Autodesk Inventor part; units mm, degrees
(part 3 of 4)
  line L522 (9.5, 12.75) -> (20, 12.75)
  line L523 (20, 12.75) -> (20, -5.25)
  line L524 (20, -5.25) -> (9.5, -5.25)
  line L525 (9.5, -5.25) -> (9.5, 12.75)
  line L526 (9.5, 17.25) -> (20, 17.25)
  line L527 (20, 17.25) -> (20, 35.25)
  line L528 (20, 35.25) -> (9.5, 35.25)
  line L529 (9.5, 35.25) -> (9.5, 17.25)
  line L530 (9.5, 57.75) -> (20, 57.75)
  line L531 (20, 57.75) -> (20, 39.75)
  line L532 (20, 39.75) -> (9.5, 39.75)
  line L533 (9.5, 39.75) -> (9.5, 57.75)
  line L534 (9.5, 62.25) -> (20, 62.25)
  line L535 (20, 62.25) -> (20, 80.25)
  line L536 (20, 80.25) -> (9.5, 80.25)
  line L537 (9.5, 80.25) -> (9.5, 62.25)
  line L538 (9.5, 117.75) -> (20, 117.75)
  line L539 (20, 117.75) -> (20, 99.75)
  line L540 (20, 99.75) -> (9.5, 99.75)
  line L541 (9.5, 99.75) -> (9.5, 117.75)
  line L542 (9.5, 84.75) -> (20, 84.75)
  line L543 (20, 84.75) -> (20, 95.25)
  line L544 (20, 95.25) -> (9.5, 95.25)
  line L545 (9.5, 95.25) -> (9.5, 84.75)
  point P0 (0, 0)
  point P1 (9.5, -64.25)
  point P2 (20, -53.75)
  point P3 (20, -49.25)
  point P4 (20, -8.75)
  point P5 (20, -4.25)
  point P6 (20, 36.25)
  point P7 (9.5, 40.75)
  point P8 (20, 51.25)
  point P9 (20, 55.75)
  point P10 (20, 96.25)
  point P11 (20, 100.75)
  point P12 (35, 27.75)
  point P13 (35, 17.25)
  point P14 (39.5, 17.25)
  point P15 (39.5, 27.75)
  point P16 (35, 42.75)
  point P17 (35, 57.75)
  point P18 (35, 72.75)
  point P19 (35, -47.25)
  point P20 (35, -77.25)
  point P21 (35, -32.25)
  point P22 (39.5, -32.25)
  point P23 (35, -17.25)
  point P24 (39.5, -17.25)
  point P25 (39.5, -12.75)
  point P26 (39.5, -2.25)
  point P27 (35, 12.75)
  point P28 (35, 2.25)
  point P29 (39.5, 2.25)
  point P30 (39.5, 12.75)
  point P31 (9.5, 99.75)
  point P32 (20, 99.75)
  point P33 (20, 102.75)
  point P34 (20, 107.25)
  point P35 (9.5, 107.25)
  point P36 (9.5, 102.75)
  point P37 (9.5, 95.25)
  point P38 (9.5, 92.25)
  point P39 (9.5, 87.75)
  point P40 (20, 84.75)
  point P41 (20, 87.75)
  point P42 (20, 92.25)
  point P43 (9.5, 80.25)
  point P44 (9.5, 77.25)
  point P45 (9.5, 72.75)
  point P46 (20, 72.75)
  point P47 (20, 77.25)
  point P48 (9.5, 39.75)
  point P49 (20, 42.75)
  point P50 (20, 47.25)
  point P51 (9.5, 47.25)
  point P52 (9.5, 42.75)
  point P53 (20, 35.25)
  point P54 (9.5, 35.25)
  point P55 (9.5, 32.25)
  point P56 (9.5, 27.75)
  point P57 (20, 27.75)
  point P58 (20, 32.25)
  point P59 (9.5, -5.25)
  point P60 (20, -5.25)
  point P61 (20, -2.25)
  point P62 (20, 2.25)
  point P63 (9.5, 2.25)
  point P64 (9.5, -2.25)
  point P65 (9.5, -9.75)
  point P66 (9.5, -12.75)
  point P67 (9.5, -17.25)
  point P68 (20, -20.25)
  point P69 (20, -17.25)
  point P70 (20, -12.75)
  point P71 (9.5, -24.75)
  point P72 (9.5, -27.75)
  point P73 (9.5, -32.25)
  point P74 (20, -32.25)
  point P75 (20, -27.75)
  point P76 (9.5, -65.25)
  point P77 (20, -62.25)
  point P78 (20, -57.75)
  point P79 (9.5, -57.75)
  point P80 (9.5, -62.25)
  point P81 (9.5, -69.75)
  point P82 (9.5, -72.75)
  point P83 (9.5, -77.25)
  point P84 (20, -77.25)
  point P85 (20, -72.75)
  dimension "d223" = 0.25
  dimension "d224" = 10.5
  dimension "d225" = 10.5
  dimension "d226" = 0.25
  dimension "d229" = 15
  dimension "d232" = 15
  dimension "d283" = 10.5
  dimension "d284" = 18
  dimension "d285" = 18
  dimension "d286" = 18
  dimension "d287" = 10.5
  dimension "d288" = 4.5
  dimension "d289" = 18
  dimension "d290" = 18
  dimension "d291" = 18
  dimension "d292" = 18
  dimension "d293" = 18
  dimension "d294" = 10.5
  dimension "d295" = 4.5
  constraints: 1088 end point, 50 parallel, 26 horizontal, 25 perpendicular, 21 point on line, 2 collinear, 1 vertical, 886 other
  measures "d223" distance between parallel lines of L4 L0
  measures "d224" distance of L0.start L0.end
  measures "d225" distance of L0.end L1.end
  measures "d226" distance between parallel lines of L5 L3
  measures "d229" distance of L0.start L6.start
  measures "d232" distance of L0.start L66.start
  measures "d283" distance of L508.end L507.end
  measures "d284" distance of L507.end L506.end
  measures "d285" distance of L510.end L511.end
  measures "d286" distance of L514.end L515.end
  measures "d287" distance of L518.end L519.end
  measures "d288" distance between parallel lines of L516 L518
  measures "d289" distance of L522.end L523.end
  measures "d290" distance of L526.end L527.end
  measures "d291" distance of L530.end L531.end
  measures "d292" distance of L534.end L535.end
  measures "d293" distance of L538.end L539.end
  measures "d294" distance of L542.end L543.end
  measures "d295" distance between parallel lines of L536 L542
extrude "Extrusion8" add sketch "Sketch21" along normal blind 1 contours L0 L1 L2 L3 | L6 L7 L8 L9 | L66 L67 L68 L69 | L70 L71 L72 L73 | L130 L131 L132 L133 | L134 L135 L136 L137 | L162 L163 L164 L165 | L166 L167 L168 L169 | L170 L171 L172 L173 | L174 L175 L176 L177 | L178 L179 L180 L181 | L182 L183 L184 L185 | L186 L187 L188 L189 | L190 L191 L192 L193 | L194 L195 L196 L197 | L198 L199 L200 L201 | L226 L227 L228 L229 | L230 L231 L232 L233 | L234 L235 L236 L237 | L238 L239 L240 L241 | L242 L243 L244 L245 | L246 L247 L248 L249 | L250 L251 L252 L253 | L254 L255 L256 L257 | L258 L259 L260 L261 | L262 L263 L264 L265 | L266 L267 L268 L269 | L268 L509 L270 L507 | L270 L271 L508 L273 | L512 L271 L272 L273 | L272 L513 L274 L511 | L274 L275 L276 L277 | L278 L279 L280 L281 | L280 L517 L282 L515 | L282 L283 L516 L285 | L518 L283 L284 L285 | L284 L521 L286 L519 | L286 L287 L520 L289 | L524 L287 L288 L289 | L288 L525 L290 L523 | L290 L291 L292 L293 | L294 L295 L296 L297 | L296 L529 L298 L527 | L298 L299 L528 L301 | L532 L299 L300 L301 | L300 L533 L302 L531 | L302 L303 L304 L305 | L306 L307 L308 L309 | L308 L537 L310 L535 | L310 L311 L536 L313 | L542 L311 L312 L313 | L312 L545 L314 L543 | L314 L315 L544 L317 | L540 L315 L316 L317 | L316 L541 L318 L539 | L318 L319 L320 L321 | L322 L323 L324 L325 | L326 L327 L328 L329 | L330 L331 L332 L333 | L333 L452 L395 L450 | L395 L396 L397 L394 | L334 L335 L336 L337 | L337 L456 L399 L454 | L399 L400 L401 L398 | L338 L339 L340 L341 | L341 L460 L403 L458 | L403 L404 L405 L402 | L342 L343 L344 L345 | L345 L464 L407 L462 | L407 L408 L409 L406 | L346 L347 L348 L349 | L349 L468 L411 L466 | L411 L412 L413 L410 | L350 L351 L352 L353 | L353 L472 L415 L470 | L415 L416 L417 L414 | L354 L355 L356 L357 | L357 L476 L419 L474 | L419 L420 L421 L418 | L358 L359 L360 L361 | L361 L480 L423 L478 | L423 L424 L425 L422 | L362 L363 L364 L365 | L365 L484 L427 L482 | L427 L428 L429 L426 | L366 L367 L368 L369 | L369 L488 L431 L486 | L431 L432 L433 L430 | L370 L371 L372 L373 | L373 L492 L435 L490 | L435 L436 L437 L434 | L374 L375 L376 L377 | L377 L496 L439 L494 | L439 L440 L441 L438 | L378 L379 L380 L381 | L381 L500 L443 L498 | L443 L444 L445 L442 | L382 L383 L384 L385 | L385 L504 L447 L502 | L447 L448 L449 L446 | L386 L387 L388 L389 | L390 L391 L392 L393
sketch "Sketch23" plane through (0, 4, 0) normal (0, 1, 0) x (1, 0, 0)
  circle A0 centre (-63.5, -131.25) radius 10.25
  line L0 (-60.5, 128.25) -> (-60.5, -128.25) projected
  line L1 (-60.5, -128.25) -> (60.5, -128.25) projected
  circle A1 centre (63.5, 131.25) radius 10.25
  circle A2 centre (63.5, -131.25) radius 10.25
  line L2 (60.5, -128.25) -> (60.5, 128.25) projected
  line L3 (60.5, 128.25) -> (-60.5, 128.25) projected
  circle A3 centre (-63.5, 131.25) radius 10.25
  circle A4 centre (-63.5, 0) radius 7.75
  circle A5 centre (63.5, 0) radius 7.75
  point P0 (0, 0)
  point P1 (-53.6989, -128.25)
  point P2 (-60.5, -121.4489)
  dimension "d338" = 20.5
  dimension "d339" = 3
  dimension "d340" = 3
  dimension "d341" = 20.5
  dimension "d342" = 3
  dimension "d343" = 3
  dimension "d344" = 20.5
  dimension "d345" = 3
  dimension "d346" = 3
  dimension "d347" = 3
  dimension "d348" = 3
  dimension "d349" = 20.5
  dimension "d350" = 15.5
  dimension "d351" = 3
  dimension "d352" = 128.25
  dimension "d353" = 15.5
  dimension "d354" = 3
  dimension "d355" = 128.25
  constraints: 6 centre point
  measures "d338" diameter of A0
  measures "d339" distance from line of L0 A0.centre
  measures "d340" distance from line of A0.centre L1
  measures "d341" diameter of A2
  measures "d342" distance from line of L2 A2.centre
  measures "d343" distance from line of L1 A2.centre
  measures "d344" diameter of A1
  measures "d345" distance from line of L3 A1.centre
  measures "d346" distance from line of L2 A1.centre
  measures "d347" distance from line of L0 A3.centre
  measures "d348" distance from line of L3 A3.centre
  measures "d349" diameter of A3
  measures "d350" diameter of A4
  measures "d351" distance from line of L0 A4.centre
  measures "d352" distance from line of L3 A4.centre
  measures "d353" diameter of A5
  measures "d354" distance from line of L2 A5.centre
  measures "d355" distance from line of L1 A5.centre
extrude "Extrusion9" cut sketch "Sketch23" against normal through all contours L1 L0 A0 | A2 L2 L1 | L1 L2 A2 | A4 L0 | L0 A4 | A5 L2 | L2 A5 | A3 L3 L0 | L0 L3 A3 | L2 L3 A1 | A1 L3 L2 picked at (-59.7398, -124.0546)
sketch "Sketch24" plane through (0, 4, 0) normal (0, 1, 0) x (1, 0, 0)
  line L0 (-52, 0.5) -> (-23, 0.5)
  line L1 (-23, 0.5) -> (-23, 29.5) construction
  line L2 (-23, 29.5) -> (-52, 29.5)
  line L3 (-52, 29.5) -> (-52, 0.5) construction
  line L4 (-52, 30.5) -> (-23, 30.5)
  line L5 (-23, 30.5) -> (-23, 59.5)
  line L6 (-23, 59.5) -> (-52, 59.5)
  line L7 (-52, 59.5) -> (-52, 30.5)
  line L8 (-52, 60.5) -> (-23, 60.5)
  line L9 (-23, 60.5) -> (-23, 89.5)
  line L10 (-23, 89.5) -> (-52, 89.5)
  line L11 (-52, 89.5) -> (-52, 60.5)
  line L12 (-52, 90.5) -> (-23, 90.5)
  line L13 (-23, 90.5) -> (-23, 119.5)
  line L14 (-23, 119.5) -> (-52, 119.5)
  line L15 (-52, 119.5) -> (-52, 90.5)
  line L16 (-60.5, 121.4489) -> (-60.5, 7.1458) projected
  line L17 (-43.5, 9) -> (-31.5, 9) construction
  line L18 (-31.5, 9) -> (-31.5, 21) construction
  line L19 (-31.5, 21) -> (-43.5, 21) construction
  line L20 (-43.5, 21) -> (-43.5, 9)
  line L21 (-43.5, 39) -> (-31.5, 39)
  line L22 (-31.5, 39) -> (-31.5, 51)
  line L23 (-31.5, 51) -> (-43.5, 51)
  line L24 (-43.5, 51) -> (-43.5, 39)
  line L25 (-43.5, 69) -> (-31.5, 69)
  line L26 (-31.5, 69) -> (-31.5, 81)
  line L27 (-31.5, 81) -> (-43.5, 81)
  line L28 (-43.5, 81) -> (-43.5, 69)
  line L29 (-43.5, 99) -> (-31.5, 99)
  line L30 (-31.5, 99) -> (-31.5, 111)
  line L31 (-31.5, 111) -> (-43.5, 111)
  line L32 (-43.5, 111) -> (-43.5, 99)
  line L33 (-49.7, 0.1) -> (-43.5, 0.1)
  line L34 (-43.5, 0.1) -> (-43.5, 26.3)
  line L35 (-43.5, 26.3) -> (-49.7, 26.3)
  line L36 (-49.7, 26.3) -> (-49.7, 0.1)
  line L37 (-49.7, 30.1) -> (-43.5, 30.1)
  line L38 (-43.5, 30.1) -> (-43.5, 56.3)
  line L39 (-43.5, 56.3) -> (-49.7, 56.3)
  line L40 (-49.7, 56.3) -> (-49.7, 30.1)
  line L41 (-49.7, 60.1) -> (-43.5, 60.1)
  line L42 (-43.5, 60.1) -> (-43.5, 86.3)
  line L43 (-43.5, 86.3) -> (-49.7, 86.3)
  line L44 (-49.7, 86.3) -> (-49.7, 60.1)
  line L45 (-49.7, 90.1) -> (-43.5, 90.1)
  line L46 (-43.5, 90.1) -> (-43.5, 116.3)
  line L47 (-43.5, 116.3) -> (-49.7, 116.3)
  line L48 (-49.7, 116.3) -> (-49.7, 90.1)
  line L49 (-31.5, 26.3) -> (-27.5, 26.3)
  line L50 (-27.5, 26.3) -> (-27.5, 6.3)
  line L51 (-27.5, 6.3) -> (-31.5, 6.3)
  line L52 (-31.5, 6.3) -> (-31.5, 26.3)
  line L53 (-31.5, 36.3) -> (-27.5, 36.3)
  line L54 (-27.5, 36.3) -> (-27.5, 56.3)
  line L55 (-27.5, 56.3) -> (-31.5, 56.3)
  line L56 (-31.5, 56.3) -> (-31.5, 36.3)
  line L57 (-31.5, 66.3) -> (-27.5, 66.3)
  line L58 (-27.5, 66.3) -> (-27.5, 86.3)
  line L59 (-27.5, 86.3) -> (-31.5, 86.3)
  line L60 (-31.5, 86.3) -> (-31.5, 66.3)
  line L61 (-31.5, 96.3) -> (-27.5, 96.3)
  line L62 (-27.5, 96.3) -> (-27.5, 116.3)
  line L63 (-27.5, 116.3) -> (-31.5, 116.3)
  line L64 (-31.5, 116.3) -> (-31.5, 96.3)
  line L65 (53.6989, 128.25) -> (-53.6989, 128.25) projected
  point P0 (0, 0)
  point P1 (-49.7, 90.5)
  point P2 (-43.5, 90.5)
  point P3 (-43.5, 111)
  point P4 (-49.7, 60.5)
  point P5 (-43.5, 60.5)
  point P6 (-43.5, 69)
  point P7 (-43.5, 81)
  point P8 (-49.7, 30.5)
  point P9 (-43.5, 30.5)
  point P10 (-43.5, 9)
  point P11 (-31.5, 39)
  point P12 (-31.5, 81)
  point P13 (-31.5, 111)
  dimension "d358" = 29
  dimension "d359" = 29
  dimension "d360" = 29
  dimension "d361" = 29
  dimension "d362" = 29
  dimension "d363" = 29
  dimension "d364" = 29
  dimension "d365" = 8.5
  dimension "d366" = 1
  dimension "d367" = 1
  dimension "d368" = 1
  dimension "d370" = 12
  dimension "d371" = 12
  dimension "d372" = 12
  dimension "d373" = 12
  dimension "d374" = 12
  dimension "d375" = 8.5
  dimension "d376" = 8.5
  dimension "d377" = 8.5
  dimension "d378" = 8.5
  dimension "d379" = 8.5
  dimension "d380" = 6.2
  dimension "d381" = 0
  dimension "d382" = 26.2
  dimension "d383" = 5.3
  dimension "d384" = 6.2
  dimension "d385" = 26.2
  dimension "d386" = 5.3
  dimension "d387" = 6.2
  dimension "d388" = 0
  dimension "d389" = 26.2
  dimension "d390" = 5.3
  dimension "d391" = 0
  dimension "d392" = 6.2
  dimension "d393" = 26.2
  dimension "d394" = 5.3
  dimension "d397" = 5.3
  dimension "d398" = 20
  dimension "d399" = 4
  dimension "d400" = 0
  dimension "d401" = 4
  dimension "d402" = 20
  dimension "d403" = 20
  dimension "d404" = 20
  dimension "d405" = 5.3
  dimension "d406" = 5.3
  dimension "d407" = 5.3
  dimension "d408" = 0
  dimension "d422" = 8.75
  constraints: 128 end point, 32 parallel, 16 horizontal, 16 perpendicular, 15 point on line
  measures "d358" distance of L0.end L1.end
  measures "d359" distance of L1.end L2.end
  measures "d360" distance of L5.end L6.end
  measures "d361" distance of L4.end L5.end
  measures "d362" distance of L8.end L9.end
  measures "d363" distance of L13.end L14.end
  measures "d364" distance of L12.end L13.end
  measures "d365" distance between parallel lines of L16 L3
  measures "d366" distance between parallel lines of L2 L4
  measures "d367" distance between parallel lines of L6 L8
  measures "d368" distance between parallel lines of L10 L12
  measures "d370" distance of L19.end L17.start
  measures "d371" distance of L18.end L19.end
  measures "d372" distance of L23.end L21.start
  measures "d373" distance of L27.end L25.start
  measures "d374" distance of L31.end L29.start
  measures "d375" distance between parallel lines of L3 L20
  measures "d376" distance between parallel lines of L2 L19
  measures "d377" distance between parallel lines of L4 L21
  measures "d378" distance between parallel lines of L8 L25
  measures "d379" distance between parallel lines of L12 L29
  measures "d380" distance of L34.end L35.end
  measures "d381" distance between parallel lines of L20 L34
  measures "d382" distance of L35.end L33.start
  measures "d383" distance between parallel lines of L19 L35
  measures "d384" distance of L46.end L47.end
  measures "d385" distance of L39.end L37.start
  measures "d386" distance between parallel lines of L39 L23
  measures "d387" distance of L38.end L39.end
  measures "d388" distance between parallel lines of L24 L38
  measures "d389" distance of L41.end L42.end
  measures "d390" distance between parallel lines of L27 L43
  measures "d391" distance between parallel lines of L28 L42
  measures "d392" distance of L42.end L43.end
  measures "d393" distance of L47.end L45.start
  measures "d394" distance between parallel lines of L31 L47
  measures "d397" distance between parallel lines of L19 L49
  measures "d398" distance of L49.end L50.end
  measures "d399" distance of L49.start L49.end
  measures "d400" distance between parallel lines of L18 L52
  measures "d401" distance of L54.end L55.end
  measures "d402" distance of L53.end L54.end
  measures "d403" distance of L57.end L58.end
  measures "d404" distance of L61.end L62.end
  measures "d405" distance between parallel lines of L31 L63
  measures "d406" distance between parallel lines of L27 L59
  measures "d407" distance between parallel lines of L23 L55
  measures "d408" distance between parallel lines of L22 L56
  measures "d422" distance between parallel lines of L65 L14
extrude "Extrusion10" add sketch "Sketch24" along normal blind 2.4 contours L36 L35 L34 L20 L0 | L0 L34 L33 L36 | L40 L39 L38 L24 L4 | L22 L56 L55 L54 L53 | L44 L43 L42 L28 L8 | L26 L60 L59 L58 L57 | L48 L47 L46 L32 L12 | L30 L64 L63 L62 L61 | L49 L50 L51 L52
sketch "Sketch25" plane through (0, 6.4, 0) normal (0, 1, 0) x (1, 0, 0)
  circle A0 centre (-46.15, 3.9) radius 1.5 projected
  circle A1 centre (-46.15, 20.6) radius 1.5 projected
  circle A2 centre (-46.15, 33.9) radius 1.5 projected
  circle A3 centre (-46.15, 50.6) radius 1.5 projected
  circle A4 centre (-46.15, 63.9) radius 1.5 projected
  circle A5 centre (-46.15, 80.6) radius 1.5 projected
  circle A6 centre (-46.15, 93.9) radius 1.5 projected
  circle A7 centre (-46.15, 110.6) radius 1.5 projected
  point P0 (0, 0)
  constraints: 8 coincident
hole "Hole1" at (-46.15, 6.4, -33.9) at (-46.15, 6.4, -50.6) at (-46.15, 6.4, -20.6) at (-46.15, 6.4, -3.9) at (-46.15, 6.4, -63.9) at (-46.15, 6.4, -80.6) at (-46.15, 6.4, -93.9) at (-46.15, 6.4, -110.6) direction (0, -1, 0) diameter 2.6 end through all
sketch "Sketch27" plane through (0, 4, 0) normal (0, 1, 0) x (1, 0, 0)
  line L0 (-43.5, 0.1) -> (-43.5, 26.3) projected
  line L1 (-27.5, 6.3) -> (-27.5, 26.3) projected
  line L2 (-43.5, 0.1) -> (-27.5, 0.1)
  line L3 (-27.5, 0.1) -> (-27.5, 6.3)
  line L4 (-27.5, 6.3) -> (-43.5, 6.3)
  line L5 (-43.5, 6.3) -> (-43.5, 0.1)
  line L6 (-43.5, 30.5) -> (-43.5, 56.3) projected
  line L7 (-27.5, 36.3) -> (-27.5, 56.3) projected
  line L8 (-43.5, 30.5) -> (-27.5, 30.5)
  line L9 (-27.5, 30.5) -> (-27.5, 36.3)
  line L10 (-27.5, 36.3) -> (-43.5, 36.3)
  line L11 (-43.5, 36.3) -> (-43.5, 30.5)
  line L12 (-43.5, 60.5) -> (-43.5, 86.3) projected
  line L13 (-31.5, 66.3) -> (-27.5, 66.3) projected
  line L14 (-43.5, 60.5) -> (-27.5, 60.5)
  line L15 (-27.5, 60.5) -> (-27.5, 66.3)
  line L16 (-27.5, 66.3) -> (-43.5, 66.3)
  line L17 (-43.5, 66.3) -> (-43.5, 60.5)
  line L18 (-43.5, 90.5) -> (-43.5, 116.3) projected
  line L19 (-31.5, 96.3) -> (-27.5, 96.3) projected
  line L20 (-43.5, 90.5) -> (-27.5, 90.5)
  line L21 (-27.5, 90.5) -> (-27.5, 96.3)
  line L22 (-27.5, 96.3) -> (-43.5, 96.3)
  line L23 (-43.5, 96.3) -> (-43.5, 90.5)
  line L24 (-60.5, 121.4489) -> (-60.5, 7.1458) projected
  line L25 (53.6989, 128.25) -> (-53.6989, 128.25) projected
  line L26 (-60.5, 120.75) -> (-19.75, 120.75)
  line L27 (-19.75, 120.75) -> (-19.75, 128.25)
  line L28 (-19.75, 128.25) -> (-60.5, 128.25)
  line L29 (-60.5, 128.25) -> (-60.5, 120.75)
  line L30 (-52.75, 123.75) -> (-22.75, 123.75) projected
  line L31 (-22.75, 123.75) -> (-22.75, 131.25) projected
  line L32 (-52.75, 131.25) -> (-22.75, 131.25) projected
  line L33 (-52.75, 123.75) -> (-52.75, 131.25) projected
  line L34 (-52.75, -131.25) -> (-22.75, -131.25) projected
  line L35 (-22.75, -131.25) -> (-22.75, -123.75) projected
  line L36 (-52.75, -123.75) -> (-22.75, -123.75) projected
  line L37 (-52.75, -131.25) -> (-52.75, -123.75) projected
  line L38 (-60.5, -7.1458) -> (-60.5, -121.4489) projected
  line L39 (-53.6989, -128.25) -> (53.6989, -128.25) projected
  line L40 (-60.5, -120.75) -> (-19.75, -120.75)
  line L41 (-19.75, -120.75) -> (-19.75, -128.25)
  line L42 (-19.75, -128.25) -> (-60.5, -128.25)
  line L43 (-60.5, -128.25) -> (-60.5, -120.75)
  point P0 (0, 0)
  point P1 (-53.6989, 128.25)
  dimension "d435" = 3
  dimension "d436" = 3
  dimension "d437" = 3
  dimension "d438" = 3
  constraints: 48 end point, 12 parallel, 6 horizontal, 6 perpendicular, 4 point on line
  measures "d435" distance between parallel lines of L27 L31
  measures "d436" distance between parallel lines of L30 L26
  measures "d437" distance between parallel lines of L40 L36
  measures "d438" distance between parallel lines of L41 L35
extrude "Extrusion11" cut sketch "Sketch27" against normal through all contours L0 L4 L3 L2 | L6 L10 L9 L8 | L12 L16 L13 L15 L14 | L18 L22 L19 L21 L20 | L29 L28 L25 L33 L30 L31 L27 L26 L24 | L25 L31 L30 L33 | L39 L42 L43 L38 L40 L41 L35 L36 L37 | L37 L36 L35 L39
sketch "Sketch28" plane through (0, 4, 0) normal (0, 1, 0) x (1, 0, 0)
  line L0 (-50.75, -88) -> (-50.75, -2) construction
  line L1 (5.25, -88) -> (-50.75, -88) construction
  line L2 (5.25, -2) -> (5.25, -88) construction
  line L3 (-50.75, -2) -> (5.25, -2) construction
  line L4 (-52.25, -1.5) -> (-52.25, -88.5)
  line L5 (-51.25, -89.5) -> (5.75, -89.5)
  line L6 (6.75, -88.5) -> (6.75, -1.5)
  line L7 (5.75, -0.5) -> (-51.25, -0.5)
  line L8 (-11, 0.5) -> (-19.5, 0.5) projected
  arc A0 (5.75, -89.5) -> (6.75, -88.5) centre (5.75, -88.5) ccw
  arc A1 (6.75, -1.5) -> (5.75, -0.5) centre (5.75, -1.5) ccw
  arc A2 (-51.25, -0.5) -> (-52.25, -1.5) centre (-51.25, -1.5) ccw
  arc A3 (-52.25, -88.5) -> (-51.25, -89.5) centre (-51.25, -88.5) ccw
  line L9 (5.25, -88) -> (-50.75, -88) projected
  point P0 (0, 0)
  dimension "d430" = 1
  dimension "d431" = 1
  constraints: 8 end point, 8 point on circle, 8 tangent, 4 centre point, 3 equal radius, 3 other
  measures "d430" distance between parallel lines of L7 L8
  measures "d431" radius of A0
extrude "Extrusion12" add sketch "Sketch28" along normal blind 20.3
sketch "Sketch30" plane through (0, 0, 0) normal (0, -1, 0) x (1, 0, 0)
  line L0 (-50.75, 2) -> (5.25, 2) construction
  line L1 (5.25, 2) -> (5.25, 88) construction
  line L2 (5.25, 88) -> (-50.75, 88) construction
  line L3 (-50.75, 88) -> (-50.75, 2) construction
  arc A0 (-51.25, 89.5) -> (-52.25, 88.5) centre (-51.25, 88.5) ccw projected
  line L4 (-51.25, 89.5) -> (5.75, 89.5) projected
  arc A1 (6.75, 88.5) -> (5.75, 89.5) centre (5.75, 88.5) ccw projected
  line L5 (6.75, 88.5) -> (6.75, 1.5) projected
  arc A2 (5.75, 0.5) -> (6.75, 1.5) centre (5.75, 1.5) ccw projected
  line L6 (5.75, 0.5) -> (-51.25, 0.5) projected
  arc A3 (-52.25, 1.5) -> (-51.25, 0.5) centre (-51.25, 1.5) ccw projected
  line L7 (-52.25, 1.5) -> (-52.25, 88.5) projected
  line L8 (-51, 1.75) -> (5.5, 1.75)
  line L9 (5.5, 1.75) -> (5.5, 88.25)
  line L10 (5.5, 88.25) -> (-51, 88.25)
  line L11 (-51, 88.25) -> (-51, 1.75)
  point P0 (0, 0)
  dimension "d439" = 1.5
  dimension "d440" = 1.5
  dimension "d441" = 1.5
  dimension "d442" = 1.5
  dimension "d443" = 0.25
  constraints: 16 end point, 4 parallel, 2 perpendicular, 1 horizontal, 3 other
  measures "d439" distance between parallel lines of L5 L1
  measures "d440" distance between parallel lines of L6 L0
  measures "d441" distance between parallel lines of L7 L3
  measures "d442" distance between parallel lines of L4 L2
  measures "d443" distance between parallel lines of L3 L11
extrude "Extrusion13" cut sketch "Sketch30" against normal through all contours L11 L10 L9 L8
sketch "Sketch31" plane through (0, 0, 0) normal (0, -1, 0) x (1, 0, 0)
  line L0 (5.25, 63) -> (-50.75, 63) projected
  line L1 (-51, 1.75) -> (-51, 88.25) projected
  line L2 (5.5, 88.25) -> (-51, 88.25) projected
  line L3 (-51, 63) -> (5.5, 63)
  line L4 (5.5, 63) -> (5.5, 88.25)
  line L5 (5.5, 88.25) -> (-51, 88.25)
  line L6 (-51, 88.25) -> (-51, 63)
  line L7 (5.5, 88.25) -> (5.5, 1.75) projected
  line L8 (5.5, 1.75) -> (-34.5, 1.75)
  line L9 (-34.5, 1.75) -> (-34.5, 5.75)
  line L10 (-34.5, 5.75) -> (5.5, 5.75)
  line L11 (5.5, 5.75) -> (5.5, 1.75)
  point P0 (0, 0)
  dimension "d446" = 4
  dimension "d447" = 40
  constraints: 16 end point, 4 parallel, 2 horizontal, 2 perpendicular, 2 point on line
  measures "d446" distance of L8.end L9.end
  measures "d447" distance between parallel lines of L7 L9
ref_plane "Work Plane1" through (-53.15, 15.8, 63) normal (0, -1, 0) x (1, 0, 0)
extrude "Extrusion14" add sketch "Sketch31" against normal up to surface (15.8 mm away)
sketch "Sketch32" plane through (0, 24.3, 0) normal (0, 1, 0) x (1, 0, 0)
  line L0 (-51.25, -89.5) -> (5.75, -89.5) projected
  arc A0 (5.75, -89.5) -> (6.75, -88.5) centre (5.75, -88.5) ccw projected
  line L1 (6.75, -88.5) -> (6.75, -1.5) projected
  arc A1 (6.75, -1.5) -> (5.75, -0.5) centre (5.75, -1.5) ccw projected
  line L2 (5.75, -0.5) -> (-51.25, -0.5) projected
  arc A2 (-51.25, -0.5) -> (-52.25, -1.5) centre (-51.25, -1.5) ccw projected
  line L3 (-52.25, -1.5) -> (-52.25, -88.5) projected
  arc A3 (-52.25, -88.5) -> (-51.25, -89.5) centre (-51.25, -88.5) ccw projected
  line L4 (5.25, -2) -> (5.25, -88) projected
  line L5 (-50.75, -2) -> (5.25, -2) projected
  line L6 (-50.75, -88) -> (-50.75, -2) projected
  line L7 (5.25, -88) -> (-50.75, -88) projected
  line L8 (-46.75, -5) -> (1.25, -5)
  line L9 (2.25, -6) -> (2.25, -84)
  line L10 (1.25, -85) -> (-46.75, -85)
  line L11 (-47.75, -84) -> (-47.75, -6)
  arc A4 (-47.75, -84) -> (-46.75, -85) centre (-46.75, -84) ccw
  arc A5 (-46.75, -5) -> (-47.75, -6) centre (-46.75, -6) ccw
  arc A6 (2.25, -6) -> (1.25, -5) centre (1.25, -6) ccw
  arc A7 (1.25, -85) -> (2.25, -84) centre (1.25, -84) ccw
  point P0 (0, 0)
  dimension "d450" = 3
  dimension "d451" = 1
  constraints: 8 end point, 8 point on circle, 8 tangent, 4 centre point, 3 equal radius, 3 other
  measures "d450" distance between parallel lines of L6 L11
  measures "d451" radius of A4
extrude "Extrusion15" add sketch "Sketch32" against normal blind 0.75 contours A3 L3 A2 L2 A1 L1 A0 L0 | L4 L7 L6 L5
sketch "Sketch33" plane through (0, 4, 0) normal (0, 1, 0) x (1, 0, 0)
  line L0 (-52, 25.75) -> (-52, 105.75) projected
  line L1 (-61.5542, 25.75) -> (-52, 25.75) projected
  line L2 (-53.9108, 105.75) -> (-52, 105.75) projected
  line L3 (-61.5542, -25.75) -> (-52, -25.75) projected
  line L4 (-52, -105.75) -> (-52, -25.75) projected
  line L5 (-61.5542, -105.75) -> (-52, -105.75) projected
  line L6 (56, -25.75) -> (40.5235, -25.75) projected
  line L7 (61.0542, -105.75) -> (51.5, -105.75) projected
  line L8 (51.5, -25.75) -> (51.5, -105.75) projected
  line L9 (51.5, 105.75) -> (51.5, 25.75) projected
  line L10 (61.0542, 105.75) -> (51.5, 105.75) projected
  line L11 (40.5235, 25.75) -> (56, 25.75) projected
  line L12 (-8, 131.25) -> (-8, 123.25) projected
  line L13 (8, 131.25) -> (8, 123.25) projected
  line L14 (-8, 123.25) -> (8, 123.25) projected
  line L15 (-8, -131.25) -> (-8, -123.25) projected
  line L16 (8, -123.25) -> (-8, -123.25) projected
  line L17 (8, -131.25) -> (8, -123.25) projected
  line L18 (60.5, 7.1458) -> (60.5, 121.4489) projected
  line L19 (60.5, -121.4489) -> (60.5, -7.1458) projected
  line L20 (-60.5, -7.1458) -> (-60.5, -120.75) projected
  point P0 (0, 0)
  point P1 (56, -65.75)
  point P2 (56, 65.75)
  point P3 (-56, 65.75)
  point P4 (-56, -65.75)
  dimension "d454" = 40
  dimension "d455" = 4.5
  dimension "d456" = 40
  dimension "d458" = 4.5
  constraints: 2 horizontal alignment, 2 vertical alignment
  measures "d454" distance from line of L11 point (56, 65.75)
  measures "d455" distance from line of L18 point (56, 65.75)
  measures "d456" distance from line of L6 point (56, -65.75)
  measures "d458" distance from line of L20 point (-56, -65.75)
hole "Hole2" at (56, 4, 65.75) at (56, 4, -65.75) at (-56, 4, -65.75) at (-56, 4, 65.75) direction (0, -1, 0) diameter 3.5 end through all counterbore diameter 6 counterbore depth 2
sketch "Sketch34" plane through (-52.25, 4, 1.5) normal (-1, 0, 0) x (0, 0, 1)
  line L0 (0.25, 11.8) -> (4.25, 11.8) projected
  line L1 (4.25, -4) -> (4.25, 11.8) projected
  line L2 (86.75, 11.8) -> (61.5, 11.8) projected
  line L3 (61.5, 11.8) -> (61.5, -4) projected
  line L4 (0.25, -4) -> (0.25, 19.55) projected
  line L5 (0.25, 19.55) -> (86.75, 19.55) projected
  line L6 (86.75, 11.8) -> (86.75, 19.55) projected
  line L7 (86.75, 19.55) -> (0.25, 19.55) projected
  line L8 (88, -4) -> (86.5, -4) projected
  line L9 (0.25, 19.55) -> (86.75, 19.55)
  line L10 (86.75, 19.55) -> (86.75, -4)
  line L11 (86.75, -4) -> (0.25, -4)
  line L12 (0.25, -4) -> (0.25, 19.55)
  line L13 (0.25, 17.8) -> (0.25, 11.8)
  line L14 (0, 20.3) -> (-1, 20.3) projected
  line L15 (-1.25, 0) -> (-1.25, -4) projected
  line L16 (-1, 0) -> (-1, -4) projected
  line L17 (5.6458, -4) -> (-8.6458, -4) projected
  point P0 (-1.5, -4)
  constraints: 10 end point, 2 parallel, 1 collinear, 1 horizontal, 1 perpendicular, 1 point on line
extrude "Extrusion16" cut sketch "Sketch34" against normal up to surface (17.75 mm away)
sketch "Sketch35" plane through (5.5, 0, 5.75) normal (-1, 0, 0) x (0, 0, 1)
  line L0 (17.25, 15.8) -> (6.75, 15.8) projected
  line L1 (17.25, 15.8) -> (17.25, 17.4) projected
  line L2 (6.75, 17.4) -> (17.25, 17.4) projected
  line L3 (6.75, 15.8) -> (6.75, 17.4) projected
  line L4 (72.25, 15.8) -> (61.75, 15.8) projected
  line L5 (72.25, 15.8) -> (72.25, 17.4) projected
  line L6 (61.75, 17.4) -> (72.25, 17.4) projected
  line L7 (61.75, 15.8) -> (61.75, 17.4) projected
  line L8 (17.5, 17.65) -> (17.5, 15.55)
  line L9 (17.5, 15.55) -> (6.5, 15.55)
  line L10 (6.5, 15.55) -> (6.5, 17.65)
  line L11 (6.5, 17.65) -> (17.5, 17.65)
  line L12 (72.5, 17.65) -> (72.5, 15.55)
  line L13 (72.5, 15.55) -> (61.5, 15.55)
  line L14 (61.5, 15.55) -> (61.5, 17.65)
  line L15 (61.5, 17.65) -> (72.5, 17.65)
  point P0 (-5.75, 0)
  dimension "d469" = 0.25
  dimension "d470" = 0.25
  constraints: 16 end point, 6 other
  measures "d469" distance between parallel lines of L2 L11
  measures "d470" distance between parallel lines of L6 L15
extrude "Extrusion17" cut sketch "Sketch35" against normal through all contours L0 L3 L2 L1 | L4 L7 L6 L5 | L8 L9 L10 L11 | L12 L13 L14 L15
sketch "Sketch38" plane through (-34.5, 0, 63) normal (-1, 0, 0) x (0, 0, 1)
  circle A0 centre (12, 10) radius 1.6 projected
  point P0 (-63, 0)
  constraints: 1 coincident
hole "Hole3" at (-34.5, 10, 75) direction (1, 0, 0) diameter 2.6 depth 6 tip angle 118
sketch "Sketch39" plane through (0, 4, 0) normal (0, 1, 0) x (1, 0, 0)
  circle A0 centre (-55.75, 10.5) radius 1.5 projected
  circle A1 centre (-55.75, 60) radius 1.5 projected
  circle A2 centre (-55.75, 109.5) radius 1.5 projected
  point P0 (0, 0)
  constraints: 3 coincident
hole "Hole4" at (-55.75, 4, -10.5) at (-55.75, 4, -109.5) at (-55.75, 4, -60) direction (0, -1, 0) diameter 2.6 depth 6 tip angle 118
sketch "Sketch40" plane through (-34.5, 0, 1.75) normal (-1, 0, 0) x (0, 0, 1)
  line L0 (5.3958, 0) -> (119, 0) projected
  line L1 (0, 0) -> (0, 15.8) projected
  line L2 (61.25, 0) -> (4, 0) projected
  line L3 (0, 9) -> (8, 9)
  line L4 (8, 9) -> (8, 0)
  line L5 (8, 0) -> (0, 0)
  line L6 (0, 0) -> (0, 9)
  point P0 (-1.75, 0)
  dimension "d496" = 8
  dimension "d497" = 9
  constraints: 8 end point, 2 parallel, 2 point on line, 1 horizontal, 1 perpendicular
  measures "d496" distance of L3.start L3.end
  measures "d497" distance between parallel lines of L0 L3
extrude "Extrusion20" add sketch "Sketch40" along normal blind 10 and the other way blind 39
sketch "Sketch41" plane through (-44.5, 0, 1.75) normal (-1, 0, 0) x (0, 0, 1)
  circle A0 centre (4.25, 7) radius 1.6 projected
  point P0 (-1.75, 0)
  constraints: 1 coincident
hole "Hole5" at (-44.5, 7, 6) direction (1, 0, 0) diameter 2.6 depth 6 tip angle 118
fillet "Fillet2" radius 0.5 16 edges at (6.4571, 24.3, 89.2071) (6.75, 24.3, 45) (6.4571, 24.3, 0.7929) (-22.75, 24.3, 0.5) (-51.9571, 24.3, 0.7929) (-52.25, 24.3, 45) (-51.9571, 24.3, 89.2071) (-22.75, 24.3, 89.5) (-47.4571, 24.3, 5.2929) (-22.75, 24.3, 5) (1.9571, 24.3, 5.2929) (2.25, 24.3, 45) (1.9571, 24.3, 84.7071) (-22.75, 24.3, 85) (-47.4571, 24.3, 84.7071) (-47.75, 24.3, 45)
sketch "Sketch42" plane through (0, 0, 0) normal (0, -1, 0) x (1, 0, 0)
  line L0 (-44.5, 1.75) -> (-52.25, 1.75) projected
  line L1 (-52.25, 1.75) -> (-52.25, 88.25) projected
  line L2 (-52.25, 88.25) -> (-34.5, 88.25) projected
  line L3 (-34.5, 88.25) -> (-34.5, 63) projected
  line L4 (-34.5, 63) -> (5.5, 63) projected
  line L5 (5.5, 63) -> (5.5, 5.75) projected
  line L6 (5.5, 5.75) -> (4.5, 5.75) projected
  line L7 (4.5, 9.75) -> (4.5, 5.75) projected
  line L8 (4.5, 9.75) -> (-44.5, 9.75) projected
  line L9 (-44.5, 1.75) -> (-44.5, 9.75) projected
  circle A0 centre (-55.75, -109.5) radius 1.3 projected
  circle A1 centre (-55.75, -10.5) radius 1.3 projected
  circle A2 centre (-55.75, -60) radius 1.3 projected
  line L10 (-60.5, -120.75) -> (-19.75, -120.75) projected
  line L11 (-19.75, -120.75) -> (-19.75, -128.25) projected
  line L12 (53.6989, -128.25) -> (-19.75, -128.25) projected
  arc A3 (60.5, -121.4489) -> (53.6989, -128.25) centre (63.5, -131.25) ccw projected
  line L13 (60.5, -7.1458) -> (60.5, -121.4489) projected
  arc A4 (60.5, 7.1458) -> (60.5, -7.1458) centre (63.5, 0) ccw projected
  line L14 (60.5, 121.4489) -> (60.5, 7.1458) projected
  arc A5 (53.6989, 128.25) -> (60.5, 121.4489) centre (63.5, 131.25) ccw projected
  line L15 (-19.75, 128.25) -> (53.6989, 128.25) projected
  line L16 (-19.75, 128.25) -> (-19.75, 120.75) projected
  line L17 (-19.75, 120.75) -> (-60.5, 120.75) projected
  line L18 (-60.5, 7.1458) -> (-60.5, 120.75) projected
  arc A6 (-60.5, -7.1458) -> (-60.5, 7.1458) centre (-63.5, 0) ccw projected
  line L19 (-60.5, -120.75) -> (-60.5, -7.1458) projected
  line L20 (-43.5, -36.3) -> (-43.5, -30.5) projected
  line L21 (-43.5, -30.5) -> (-27.5, -30.5) projected
  line L22 (-27.5, -30.5) -> (-27.5, -36.3) projected
  line L23 (-27.5, -36.3) -> (-43.5, -36.3) projected
  line L24 (-43.5, -6.3) -> (-43.5, -0.1) projected
  line L25 (-43.5, -0.1) -> (-27.5, -0.1) projected
  line L26 (-27.5, -0.1) -> (-27.5, -6.3) projected
  line L27 (-27.5, -6.3) -> (-43.5, -6.3) projected
  line L28 (-43.5, -66.3) -> (-43.5, -60.5) projected
  line L29 (-43.5, -60.5) -> (-27.5, -60.5) projected
  line L30 (-27.5, -60.5) -> (-27.5, -66.3) projected
  line L31 (-27.5, -66.3) -> (-43.5, -66.3) projected
  line L32 (-43.5, -96.3) -> (-43.5, -90.5) projected
  line L33 (-43.5, -90.5) -> (-27.5, -90.5) projected
  line L34 (-27.5, -90.5) -> (-27.5, -96.3) projected
  line L35 (-27.5, -96.3) -> (-43.5, -96.3) projected
  circle A7 centre (-46.15, -93.9) radius 1.3 projected
  circle A8 centre (-46.15, -63.9) radius 1.3 projected
  circle A9 centre (-46.15, -20.6) radius 1.3 projected
  circle A10 centre (-46.15, -33.9) radius 1.3 projected
  circle A11 centre (-46.15, -50.6) radius 1.3 projected
  circle A12 centre (-46.15, -3.9) radius 1.3 projected
  circle A13 centre (-46.15, -80.6) radius 1.3 projected
  circle A14 centre (-46.15, -110.6) radius 1.3 projected
  line L36 (21.75, 29.75) -> (20.25, 29.75) projected
  line L37 (20.25, 29.75) -> (20.25, 37.75) projected
  line L38 (20.25, 37.75) -> (21.75, 37.75) projected
  line L39 (21.75, 37.75) -> (21.75, 29.75) projected
  line L40 (20.25, -44.75) -> (21.75, -44.75) projected
  line L41 (21.75, -44.75) -> (21.75, -52.75) projected
  line L42 (21.75, -52.75) -> (20.25, -52.75) projected
  line L43 (20.25, -52.75) -> (20.25, -44.75) projected
  line L44 (51.75, -101.5) -> (50.25, -101.5) projected
  line L45 (50.25, -101.5) -> (50.25, -93.5) projected
  line L46 (50.25, -93.5) -> (51.75, -93.5) projected
  line L47 (51.75, -93.5) -> (51.75, -101.5) projected
  line L48 (51.75, -41.5) -> (50.25, -41.5) projected
  line L49 (50.25, -41.5) -> (50.25, -33.5) projected
  line L50 (50.25, -33.5) -> (51.75, -33.5) projected
  line L51 (51.75, -33.5) -> (51.75, -41.5) projected
  line L52 (51.75, 78.5) -> (50.25, 78.5) projected
  line L53 (50.25, 78.5) -> (50.25, 86.5) projected
  line L54 (50.25, 86.5) -> (51.75, 86.5) projected
  line L55 (51.75, 86.5) -> (51.75, 78.5) projected
  line L56 (51.75, 33.5) -> (50.25, 33.5) projected
  line L57 (50.25, 33.5) -> (50.25, 41.5) projected
  line L58 (50.25, 41.5) -> (51.75, 41.5) projected
  line L59 (51.75, 41.5) -> (51.75, 33.5) projected
  line L60 (-8.25, -116.5) -> (-9.75, -116.5) projected
  line L61 (-9.75, -116.5) -> (-9.75, -108.5) projected
  line L62 (-9.75, -108.5) -> (-8.25, -108.5) projected
  line L63 (-8.25, -108.5) -> (-8.25, -116.5) projected
  line L64 (6.75, -71.5) -> (5.25, -71.5) projected
  line L65 (5.25, -71.5) -> (5.25, -63.5) projected
  line L66 (5.25, -63.5) -> (6.75, -63.5) projected
  line L67 (6.75, -63.5) -> (6.75, -71.5) projected
  line L68 (6.75, -41.5) -> (5.25, -41.5) projected
  line L69 (5.25, -41.5) -> (5.25, -33.5) projected
  line L70 (5.25, -33.5) -> (6.75, -33.5) projected
  line L71 (6.75, -33.5) -> (6.75, -41.5) projected
  line L72 (6.75, -56.5) -> (5.25, -56.5) projected
  line L73 (5.25, -56.5) -> (5.25, -48.5) projected
  line L74 (5.25, -48.5) -> (6.75, -48.5) projected
  line L75 (6.75, -48.5) -> (6.75, -56.5) projected
  line L76 (-8.25, 108.5) -> (-9.75, 108.5) projected
  line L77 (-9.75, 108.5) -> (-9.75, 116.5) projected
  line L78 (-9.75, 116.5) -> (-8.25, 116.5) projected
  line L79 (-8.25, 116.5) -> (-8.25, 108.5) projected
  line L80 (51.75, 108.5) -> (50.25, 108.5) projected
  line L81 (50.25, 108.5) -> (50.25, 116.5) projected
  line L82 (50.25, 116.5) -> (51.75, 116.5) projected
  line L83 (51.75, 116.5) -> (51.75, 108.5) projected
  line L84 (6.75, 93.5) -> (5.25, 93.5) projected
  line L85 (5.25, 93.5) -> (5.25, 101.5) projected
  line L86 (5.25, 101.5) -> (6.75, 101.5) projected
  line L87 (6.75, 101.5) -> (6.75, 93.5) projected
  line L88 (51.75, 93.5) -> (50.25, 93.5) projected
  line L89 (50.25, 93.5) -> (50.25, 101.5) projected
  line L90 (50.25, 101.5) -> (51.75, 101.5) projected
  line L91 (51.75, 101.5) -> (51.75, 93.5) projected
  line L92 (-8.25, 93.5) -> (-9.75, 93.5) projected
  line L93 (-9.75, 93.5) -> (-9.75, 101.5) projected
  line L94 (-9.75, 101.5) -> (-8.25, 101.5) projected
  line L95 (-8.25, 101.5) -> (-8.25, 93.5) projected
  line L96 (36.75, 108.5) -> (35.25, 108.5) projected
  line L97 (35.25, 108.5) -> (35.25, 116.5) projected
  line L98 (35.25, 116.5) -> (36.75, 116.5) projected
  line L99 (36.75, 116.5) -> (36.75, 108.5) projected
  line L100 (-23.25, 108.5) -> (-24.75, 108.5) projected
  line L101 (-24.75, 108.5) -> (-24.75, 116.5) projected
  line L102 (-24.75, 116.5) -> (-23.25, 116.5) projected
  line L103 (-23.25, 116.5) -> (-23.25, 108.5) projected
  line L104 (-8.25, -11.5) -> (-9.75, -11.5) projected
  line L105 (-9.75, -11.5) -> (-9.75, -3.5) projected
  line L106 (-9.75, -3.5) -> (-8.25, -3.5) projected
  line L107 (-8.25, -3.5) -> (-8.25, -11.5) projected
  line L108 (-8.25, -56.5) -> (-9.75, -56.5) projected
  line L109 (-9.75, -56.5) -> (-9.75, -48.5) projected
  line L110 (-9.75, -48.5) -> (-8.25, -48.5) projected
  line L111 (-8.25, -48.5) -> (-8.25, -56.5) projected
  line L112 (-8.25, -86.5) -> (-9.75, -86.5) projected
  line L113 (-9.75, -86.5) -> (-9.75, -78.5) projected
  line L114 (-9.75, -78.5) -> (-8.25, -78.5) projected
  line L115 (-8.25, -78.5) -> (-8.25, -86.5) projected
  line L116 (6.75, -116.5) -> (5.25, -116.5) projected
  line L117 (5.25, -116.5) -> (5.25, -108.5) projected
  line L118 (5.25, -108.5) -> (6.75, -108.5) projected
  line L119 (6.75, -108.5) -> (6.75, -116.5) projected
  line L120 (51.75, 48.5) -> (50.25, 48.5) projected
  line L121 (50.25, 48.5) -> (50.25, 56.5) projected
  line L122 (50.25, 56.5) -> (51.75, 56.5) projected
  line L123 (51.75, 56.5) -> (51.75, 48.5) projected
  line L124 (51.75, -11.5) -> (50.25, -11.5) projected
  line L125 (50.25, -11.5) -> (50.25, -3.5) projected
  line L126 (50.25, -3.5) -> (51.75, -3.5) projected
  line L127 (51.75, -3.5) -> (51.75, -11.5) projected
  line L128 (51.75, -86.5) -> (50.25, -86.5) projected
  line L129 (50.25, -86.5) -> (50.25, -78.5) projected
  line L130 (50.25, -78.5) -> (51.75, -78.5) projected
  line L131 (51.75, -78.5) -> (51.75, -86.5) projected
  line L132 (20.25, -104.75) -> (21.75, -104.75) projected
  line L133 (21.75, -104.75) -> (21.75, -112.75) projected
  line L134 (21.75, -112.75) -> (20.25, -112.75) projected
  line L135 (20.25, -112.75) -> (20.25, -104.75) projected
  line L136 (21.75, -30.25) -> (20.25, -30.25) projected
  line L137 (20.25, -30.25) -> (20.25, -22.25) projected
  line L138 (20.25, -22.25) -> (21.75, -22.25) projected
  line L139 (21.75, -22.25) -> (21.75, -30.25) projected
  line L140 (20.25, 60.25) -> (21.75, 60.25) projected
  line L141 (21.75, 60.25) -> (21.75, 52.25) projected
  line L142 (21.75, 52.25) -> (20.25, 52.25) projected
  line L143 (20.25, 52.25) -> (20.25, 60.25) projected
  line L144 (21.75, 11) -> (20.25, 11) projected
  line L145 (20.25, 11) -> (20.25, 19) projected
  line L146 (20.25, 19) -> (21.75, 19) projected
  line L147 (21.75, 19) -> (21.75, 11) projected
  line L148 (21.75, -75.25) -> (20.25, -75.25) projected
  line L149 (20.25, -75.25) -> (20.25, -67.25) projected
  line L150 (20.25, -67.25) -> (21.75, -67.25) projected
  line L151 (21.75, -67.25) -> (21.75, -75.25) projected
  line L152 (51.75, -71.5) -> (50.25, -71.5) projected
  line L153 (50.25, -71.5) -> (50.25, -63.5) projected
  line L154 (50.25, -63.5) -> (51.75, -63.5) projected
  line L155 (51.75, -63.5) -> (51.75, -71.5) projected
  line L156 (51.75, -26.5) -> (50.25, -26.5) projected
  line L157 (50.25, -26.5) -> (50.25, -18.5) projected
  line L158 (50.25, -18.5) -> (51.75, -18.5) projected
  line L159 (51.75, -18.5) -> (51.75, -26.5) projected
  line L160 (51.75, 63.5) -> (50.25, 63.5) projected
  line L161 (50.25, 63.5) -> (50.25, 71.5) projected
  line L162 (50.25, 71.5) -> (51.75, 71.5) projected
  line L163 (51.75, 71.5) -> (51.75, 63.5) projected
  line L164 (51.75, 18.5) -> (50.25, 18.5) projected
  line L165 (50.25, 18.5) -> (50.25, 26.5) projected
  line L166 (50.25, 26.5) -> (51.75, 26.5) projected
  line L167 (51.75, 26.5) -> (51.75, 18.5) projected
  line L168 (6.75, -101.5) -> (5.25, -101.5) projected
  line L169 (5.25, -101.5) -> (5.25, -93.5) projected
  line L170 (5.25, -93.5) -> (6.75, -93.5) projected
  line L171 (6.75, -93.5) -> (6.75, -101.5) projected
  line L172 (-8.25, -101.5) -> (-9.75, -101.5) projected
  line L173 (-9.75, -101.5) -> (-9.75, -93.5) projected
  line L174 (-9.75, -93.5) -> (-8.25, -93.5) projected
  line L175 (-8.25, -93.5) -> (-8.25, -101.5) projected
  line L176 (6.75, -26.5) -> (5.25, -26.5) projected
  line L177 (5.25, -26.5) -> (5.25, -18.5) projected
  line L178 (5.25, -18.5) -> (6.75, -18.5) projected
  line L179 (6.75, -18.5) -> (6.75, -26.5) projected
  line L180 (-8.25, -41.5) -> (-9.75, -41.5) projected
  line L181 (-9.75, -41.5) -> (-9.75, -33.5) projected
  line L182 (-9.75, -33.5) -> (-8.25, -33.5) projected
  line L183 (-8.25, -33.5) -> (-8.25, -41.5) projected
  line L184 (6.75, 108.5) -> (5.25, 108.5) projected
  line L185 (5.25, 108.5) -> (5.25, 116.5) projected
  line L186 (5.25, 116.5) -> (6.75, 116.5) projected
  line L187 (6.75, 116.5) -> (6.75, 108.5) projected
  line L188 (-38.25, 93.5) -> (-39.75, 93.5) projected
  line L189 (-39.75, 93.5) -> (-39.75, 101.5) projected
  line L190 (-39.75, 101.5) -> (-38.25, 101.5) projected
  line L191 (-38.25, 101.5) -> (-38.25, 93.5) projected
  line L192 (21.75, 93.5) -> (20.25, 93.5) projected
  line L193 (20.25, 93.5) -> (20.25, 101.5) projected
  line L194 (20.25, 101.5) -> (21.75, 101.5) projected
  line L195 (21.75, 101.5) -> (21.75, 93.5) projected
  line L196 (36.75, 93.5) -> (35.25, 93.5) projected
  line L197 (35.25, 93.5) -> (35.25, 101.5) projected
  line L198 (35.25, 101.5) -> (36.75, 101.5) projected
  line L199 (36.75, 101.5) -> (36.75, 93.5) projected
  line L200 (-23.25, 93.5) -> (-24.75, 93.5) projected
  line L201 (-24.75, 93.5) -> (-24.75, 101.5) projected
  line L202 (-24.75, 101.5) -> (-23.25, 101.5) projected
  line L203 (-23.25, 101.5) -> (-23.25, 93.5) projected
  line L204 (21.75, 108.5) -> (20.25, 108.5) projected
  line L205 (20.25, 108.5) -> (20.25, 116.5) projected
  line L206 (20.25, 116.5) -> (21.75, 116.5) projected
  line L207 (21.75, 116.5) -> (21.75, 108.5) projected
  line L208 (-38.25, 108.5) -> (-39.75, 108.5) projected
  line L209 (-39.75, 108.5) -> (-39.75, 116.5) projected
  line L210 (-39.75, 116.5) -> (-38.25, 116.5) projected
  line L211 (-38.25, 116.5) -> (-38.25, 108.5) projected
  line L212 (-8.25, -26.5) -> (-9.75, -26.5) projected
  line L213 (-9.75, -26.5) -> (-9.75, -18.5) projected
  line L214 (-9.75, -18.5) -> (-8.25, -18.5) projected
  line L215 (-8.25, -18.5) -> (-8.25, -26.5) projected
  line L216 (-8.25, -71.5) -> (-9.75, -71.5) projected
  line L217 (-9.75, -71.5) -> (-9.75, -63.5) projected
  line L218 (-9.75, -63.5) -> (-8.25, -63.5) projected
  line L219 (-8.25, -63.5) -> (-8.25, -71.5) projected
  line L220 (6.75, -86.5) -> (5.25, -86.5) projected
  line L221 (5.25, -86.5) -> (5.25, -78.5) projected
  line L222 (5.25, -78.5) -> (6.75, -78.5) projected
  line L223 (6.75, -78.5) -> (6.75, -86.5) projected
  line L224 (6.75, -11.5) -> (5.25, -11.5) projected
  line L225 (5.25, -11.5) -> (5.25, -3.5) projected
  line L226 (5.25, -3.5) -> (6.75, -3.5) projected
  line L227 (6.75, -3.5) -> (6.75, -11.5) projected
  line L228 (51.75, 3.5) -> (50.25, 3.5) projected
  line L229 (50.25, 3.5) -> (50.25, 11.5) projected
  line L230 (50.25, 11.5) -> (51.75, 11.5) projected
  line L231 (51.75, 11.5) -> (51.75, 3.5) projected
  line L232 (51.75, -56.5) -> (50.25, -56.5) projected
  line L233 (50.25, -56.5) -> (50.25, -48.5) projected
  line L234 (50.25, -48.5) -> (51.75, -48.5) projected
  line L235 (51.75, -48.5) -> (51.75, -56.5) projected
  line L236 (51.75, -116.5) -> (50.25, -116.5) projected
  line L237 (50.25, -116.5) -> (50.25, -108.5) projected
  line L238 (50.25, -108.5) -> (51.75, -108.5) projected
  line L239 (51.75, -108.5) -> (51.75, -116.5) projected
  line L240 (21.75, -94) -> (20.25, -94) projected
  line L241 (20.25, -94) -> (20.25, -86) projected
  line L242 (20.25, -86) -> (21.75, -86) projected
  line L243 (21.75, -86) -> (21.75, -94) projected
  line L244 (20.25, 0.25) -> (21.75, 0.25) projected
  line L245 (21.75, 0.25) -> (21.75, -7.75) projected
  line L246 (21.75, -7.75) -> (20.25, -7.75) projected
  line L247 (20.25, -7.75) -> (20.25, 0.25) projected
  line L248 (21.75, 74.75) -> (20.25, 74.75) projected
  line L249 (20.25, 74.75) -> (20.25, 82.75) projected
  line L250 (20.25, 82.75) -> (21.75, 82.75) projected
  line L251 (21.75, 82.75) -> (21.75, 74.75) projected
  line L252 (19, 45.5) -> (10.5, 45.5) projected
  line L253 (10.5, 45.5) -> (10.5, 47) projected
  line L254 (10.5, 47) -> (19, 47) projected
  line L255 (19, 47) -> (19, 45.5) projected
  line L256 (19, 8) -> (10.5, 8) projected
  line L257 (10.5, 8) -> (10.5, 9.5) projected
  line L258 (10.5, 9.5) -> (19, 9.5) projected
  line L259 (19, 9.5) -> (19, 8) projected
  line L260 (19, -59.5) -> (10.5, -59.5) projected
  line L261 (10.5, -59.5) -> (10.5, -58) projected
  line L262 (10.5, -58) -> (19, -58) projected
  line L263 (19, -58) -> (19, -59.5) projected
  line L264 (19, -97) -> (10.5, -97) projected
  line L265 (10.5, -97) -> (10.5, -95.5) projected
  line L266 (10.5, -95.5) -> (19, -95.5) projected
  line L267 (19, -95.5) -> (19, -97) projected
  line L268 (-41, 103) -> (-49.5, 103) projected
  line L269 (-49.5, 103) -> (-49.5, 104.5) projected
  line L270 (-49.5, 104.5) -> (-41, 104.5) projected
  line L271 (-41, 104.5) -> (-41, 103) projected
  line L272 (-26, 90.5) -> (-34.5, 90.5) projected
  line L273 (-34.5, 90.5) -> (-34.5, 92) projected
  line L274 (-34.5, 92) -> (-26, 92) projected
  line L275 (-26, 92) -> (-26, 90.5) projected
  line L276 (-11, 90.5) -> (-19.5, 90.5) projected
  line L277 (-19.5, 90.5) -> (-19.5, 92) projected
  line L278 (-19.5, 92) -> (-11, 92) projected
  line L279 (-11, 92) -> (-11, 90.5) projected
  line L280 (4, 90.5) -> (-4.5, 90.5) projected
  line L281 (-4.5, 90.5) -> (-4.5, 92) projected
  line L282 (-4.5, 92) -> (4, 92) projected
  line L283 (4, 92) -> (4, 90.5) projected
  line L284 (49, 105.5) -> (40.5, 105.5) projected
  line L285 (40.5, 105.5) -> (40.5, 107) projected
  line L286 (40.5, 107) -> (49, 107) projected
  line L287 (49, 107) -> (49, 105.5) projected
  line L288 (34, 105.5) -> (25.5, 105.5) projected
  line L289 (25.5, 105.5) -> (25.5, 107) projected
  line L290 (25.5, 107) -> (34, 107) projected
  line L291 (34, 107) -> (34, 105.5) projected
  line L292 (19, 105.5) -> (10.5, 105.5) projected
  line L293 (10.5, 105.5) -> (10.5, 107) projected
  line L294 (10.5, 107) -> (19, 107) projected
  line L295 (19, 107) -> (19, 105.5) projected
  line L296 (49, 15.5) -> (40.5, 15.5) projected
  line L297 (40.5, 15.5) -> (40.5, 17) projected
  line L298 (40.5, 17) -> (49, 17) projected
  line L299 (49, 17) -> (49, 15.5) projected
  line L300 (34, 13) -> (25.5, 13) projected
  line L301 (25.5, 13) -> (25.5, 14.5) projected
  line L302 (25.5, 14.5) -> (34, 14.5) projected
  line L303 (34, 14.5) -> (34, 13) projected
  line L304 (34, 43) -> (25.5, 43) projected
  line L305 (25.5, 43) -> (25.5, 44.5) projected
  line L306 (25.5, 44.5) -> (34, 44.5) projected
  line L307 (34, 44.5) -> (34, 43) projected
  line L308 (34, 0.5) -> (25.5, 0.5) projected
  line L309 (25.5, 0.5) -> (25.5, 2) projected
  line L310 (25.5, 2) -> (34, 2) projected
  line L311 (34, 2) -> (34, 0.5) projected
  line L312 (49, 60.5) -> (40.5, 60.5) projected
  line L313 (40.5, 60.5) -> (40.5, 62) projected
  line L314 (40.5, 62) -> (49, 62) projected
  line L315 (49, 62) -> (49, 60.5) projected
  line L316 (34, 73) -> (25.5, 73) projected
  line L317 (25.5, 73) -> (25.5, 74.5) projected
  line L318 (25.5, 74.5) -> (34, 74.5) projected
  line L319 (34, 74.5) -> (34, 73) projected
  line L320 (49, -59.5) -> (40.5, -59.5) projected
  line L321 (40.5, -59.5) -> (40.5, -58) projected
  line L322 (40.5, -58) -> (49, -58) projected
  line L323 (49, -58) -> (49, -59.5) projected
  line L324 (49, -29.5) -> (40.5, -29.5) projected
  line L325 (40.5, -29.5) -> (40.5, -28) projected
  line L326 (40.5, -28) -> (49, -28) projected
  line L327 (49, -28) -> (49, -29.5) projected
  line L328 (34, -59.5) -> (25.5, -59.5) projected
  line L329 (25.5, -59.5) -> (25.5, -58) projected
  line L330 (25.5, -58) -> (34, -58) projected
  line L331 (34, -58) -> (34, -59.5) projected
  line L332 (34, -17) -> (25.5, -17) projected
  line L333 (25.5, -17) -> (25.5, -15.5) projected
  line L334 (25.5, -15.5) -> (34, -15.5) projected
  line L335 (34, -15.5) -> (34, -17) projected
  line L336 (49, -107) -> (40.5, -107) projected
  line L337 (40.5, -107) -> (40.5, -105.5) projected
  line L338 (40.5, -105.5) -> (49, -105.5) projected
  line L339 (49, -105.5) -> (49, -107) projected
  line L340 (49, -74.5) -> (40.5, -74.5) projected
  line L341 (40.5, -74.5) -> (40.5, -73) projected
  line L342 (40.5, -73) -> (49, -73) projected
  line L343 (49, -73) -> (49, -74.5) projected
  line L344 (34, -77) -> (25.5, -77) projected
  line L345 (25.5, -77) -> (25.5, -75.5) projected
  line L346 (25.5, -75.5) -> (34, -75.5) projected
  line L347 (34, -75.5) -> (34, -77) projected
  line L348 (49, -92) -> (40.5, -92) projected
  line L349 (40.5, -92) -> (40.5, -90.5) projected
  line L350 (40.5, -90.5) -> (49, -90.5) projected
  line L351 (49, -90.5) -> (49, -92) projected
  line L352 (-11, -14.5) -> (-19.5, -14.5) projected
  line L353 (-19.5, -14.5) -> (-19.5, -13) projected
  line L354 (-19.5, -13) -> (-11, -13) projected
  line L355 (-11, -13) -> (-11, -14.5) projected
  line L356 (-11, -47) -> (-19.5, -47) projected
  line L357 (-19.5, -47) -> (-19.5, -45.5) projected
  line L358 (-19.5, -45.5) -> (-11, -45.5) projected
  line L359 (-11, -45.5) -> (-11, -47) projected
  line L360 (4, -17) -> (-4.5, -17) projected
  line L361 (-4.5, -17) -> (-4.5, -15.5) projected
  line L362 (-4.5, -15.5) -> (4, -15.5) projected
  line L363 (4, -15.5) -> (4, -17) projected
  line L364 (4, -32) -> (-4.5, -32) projected
  line L365 (-4.5, -32) -> (-4.5, -30.5) projected
  line L366 (-4.5, -30.5) -> (4, -30.5) projected
  line L367 (4, -30.5) -> (4, -32) projected
  line L368 (-11, -74.5) -> (-19.5, -74.5) projected
  line L369 (-19.5, -74.5) -> (-19.5, -73) projected
  line L370 (-19.5, -73) -> (-11, -73) projected
  line L371 (-11, -73) -> (-11, -74.5) projected
  line L372 (-11, -104.5) -> (-19.5, -104.5) projected
  line L373 (-19.5, -104.5) -> (-19.5, -103) projected
  line L374 (-19.5, -103) -> (-11, -103) projected
  line L375 (-11, -103) -> (-11, -104.5) projected
  line L376 (4, -92) -> (-4.5, -92) projected
  line L377 (-4.5, -92) -> (-4.5, -90.5) projected
  line L378 (-4.5, -90.5) -> (4, -90.5) projected
  line L379 (4, -90.5) -> (4, -92) projected
  line L380 (4, -107) -> (-4.5, -107) projected
  line L381 (-4.5, -107) -> (-4.5, -105.5) projected
  line L382 (-4.5, -105.5) -> (4, -105.5) projected
  line L383 (4, -105.5) -> (4, -107) projected
  line L384 (19, -17) -> (10.5, -17) projected
  line L385 (10.5, -17) -> (10.5, -15.5) projected
  line L386 (10.5, -15.5) -> (19, -15.5) projected
  line L387 (19, -15.5) -> (19, -17) projected
  line L388 (19, -14.5) -> (10.5, -14.5) projected
  line L389 (10.5, -14.5) -> (10.5, -13) projected
  line L390 (10.5, -13) -> (19, -13) projected
  line L391 (19, -13) -> (19, -14.5) projected
  line L392 (4, -74.5) -> (-4.5, -74.5) projected
  line L393 (-4.5, -74.5) -> (-4.5, -73) projected
  line L394 (-4.5, -73) -> (4, -73) projected
  line L395 (4, -73) -> (4, -74.5) projected
  line L396 (4, -119.5) -> (-4.5, -119.5) projected
  line L397 (-4.5, -119.5) -> (-4.5, -118) projected
  line L398 (-4.5, -118) -> (4, -118) projected
  line L399 (4, -118) -> (4, -119.5) projected
  line L400 (-11, -92) -> (-19.5, -92) projected
  line L401 (-19.5, -92) -> (-19.5, -90.5) projected
  line L402 (-19.5, -90.5) -> (-11, -90.5) projected
  line L403 (-11, -90.5) -> (-11, -92) projected
  line L404 (4, -47) -> (-4.5, -47) projected
  line L405 (-4.5, -47) -> (-4.5, -45.5) projected
  line L406 (-4.5, -45.5) -> (4, -45.5) projected
  line L407 (4, -45.5) -> (4, -47) projected
  line L408 (4, -44.5) -> (-4.5, -44.5) projected
  line L409 (-4.5, -44.5) -> (-4.5, -43) projected
  line L410 (-4.5, -43) -> (4, -43) projected
  line L411 (4, -43) -> (4, -44.5) projected
  line L412 (4, -14.5) -> (-4.5, -14.5) projected
  line L413 (-4.5, -14.5) -> (-4.5, -13) projected
  line L414 (-4.5, -13) -> (4, -13) projected
  line L415 (4, -13) -> (4, -14.5) projected
  line L416 (-11, -32) -> (-19.5, -32) projected
  line L417 (-19.5, -32) -> (-19.5, -30.5) projected
  line L418 (-19.5, -30.5) -> (-11, -30.5) projected
  line L419 (-11, -30.5) -> (-11, -32) projected
  line L420 (4, -2) -> (-4.5, -2) projected
  line L421 (-4.5, -2) -> (-4.5, -0.5) projected
  line L422 (-4.5, -0.5) -> (4, -0.5) projected
  line L423 (4, -0.5) -> (4, -2) projected
  line L424 (34, -107) -> (25.5, -107) projected
  line L425 (25.5, -107) -> (25.5, -105.5) projected
  line L426 (25.5, -105.5) -> (34, -105.5) projected
  line L427 (34, -105.5) -> (34, -107) projected
  line L428 (34, -89.5) -> (25.5, -89.5) projected
  line L429 (25.5, -89.5) -> (25.5, -88) projected
  line L430 (25.5, -88) -> (34, -88) projected
  line L431 (34, -88) -> (34, -89.5) projected
  line L432 (49, -77) -> (40.5, -77) projected
  line L433 (40.5, -77) -> (40.5, -75.5) projected
  line L434 (40.5, -75.5) -> (49, -75.5) projected
  line L435 (49, -75.5) -> (49, -77) projected
  line L436 (49, -119.5) -> (40.5, -119.5) projected
  line L437 (40.5, -119.5) -> (40.5, -118) projected
  line L438 (40.5, -118) -> (49, -118) projected
  line L439 (49, -118) -> (49, -119.5) projected
  line L440 (34, -32) -> (25.5, -32) projected
  line L441 (25.5, -32) -> (25.5, -30.5) projected
  line L442 (25.5, -30.5) -> (34, -30.5) projected
  line L443 (34, -30.5) -> (34, -32) projected